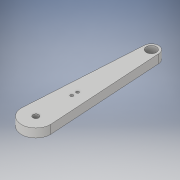
# Autodesk Inventor part: Servo_Arm
Saved by Autodesk Inventor 2019 (Build 230136000, 136)
## iProperties
Created: 2019-09-26
Part Number: Servo_Arm
Material: Generic
Document SubType Name: Modeling
Designer: Jorian Bruslind
Density: 1 g/cm^3
Appearance: Default
Author: Jorian Bruslind
Autodesk Inventor part; units mm, degrees
ref_plane "YZ Plane" through (0, 0, 0) normal (1, 0, 0) x (0, 1, 0)
ref_plane "XZ Plane" through (0, 0, 0) normal (0, 1, 0) x (-1, 0, 0)
ref_plane "XY Plane" through (0, 0, 0) normal (0, 0, 1) x (1, 0, 0)
sketch "Sketch1" plane through (0, 0, 0) normal (0, 1, 0) x (-1, 0, 0)
  circle A0 centre (0, 0) radius 5
  line L0 (0, 0) -> (0, -40)
  circle A1 centre (0, -40) radius 1.75
  circle A2 centre (0, -40) radius 2.5
  line L1 (0, -40) -> (2.5, -40)
  line L2 (0, 0) -> (5, 0)
  line L3 (5, 0) -> (2.5, -40)
  line L4 (0, 0) -> (-5, 0)
  line L5 (0, -40) -> (-2.5, -40)
  line L6 (-5, 0) -> (-2.5, -40)
  dimension "d0" = 10
  dimension "d1" = 40
  dimension "d2" = 3.5
  dimension "d3" = 5
  constraints: 14 end point, 4 point on circle, 3 centre point, 3 coincident, 2 horizontal, 2 parallel, 1 vertical
  measures "d0" diameter of A0
  measures "d1" distance of L0.start L0.end
  measures "d2" diameter of A1
  measures "d3" diameter of A2
extrude "Extrusion1" add sketch "Sketch1" along normal blind 3 contours L2 L4 A0 | L3 A0 L0 L2 | L4 L0 A0 L6 | L3 A2 L0 A0 | A0 L0 A2 L6 | L1 A1 L0 A2 | A2 L5 A1 L1 | A2 L0 A1 L5 | L1 L0 A1 | A1 L5 L1 | A1 L0 L5
sketch "Sketch2" plane through (0, 3, 0) normal (0, 1, 0) x (1, 0, 0)
  arc A0 (2.5, 40) -> (-2.5, 40) centre (0, 40) ccw projected
  circle A1 centre (0, 40) radius 1.75
  point P0 (0, 0)
  dimension "d6" = 3.5
  constraints: 1 centre point, 1 coincident
  measures "d6" diameter of A1
extrude "Extrusion2" cut sketch "Sketch2" against normal blind 5
sketch "Sketch4" plane through (0, 0, 0) normal (0, -1, 0) x (1, 0, 0)
  circle A0 centre (0, 0) radius 4
  line L0 (0, 0) -> (0, -14.45)
  circle A1 centre (0, -14.45) radius 2.5
  line L1 (0, 0) -> (-4, 0)
  line L2 (0, -14.45) -> (-2.5, -14.45)
  line L3 (0, -14.45) -> (2.5, -14.45)
  line L4 (0, 0) -> (4, 0)
  line L5 (2.5, -14.45) -> (13.578, -14.45) construction
  line L6 (2.5, -14.45) -> (3.0315, -2.6097)
  line L7 (2.5, -14.45) -> (14.3523, -14.45) construction
  line L8 (-2.5, -14.45) -> (-3.0325, -2.6084)
  line L9 (-2.5, -14.45) -> (9.3536, -14.45) construction
  dimension "d12" = 8
  dimension "d13" = 14.45
  dimension "d14" = 5
  dimension "d16" = 87.43
  dimension "d17" = 92.575
  constraints: 20 end point, 6 point on circle, 4 horizontal, 2 centre point, 2 coincident, 2 equal length, 2 point on line, 1 parallel, 1 vertical
  measures "d12" diameter of A0
  measures "d13" distance of L0.start L0.end
  measures "d14" diameter of A1
  measures "d16" angle of L7 L6
  measures "d17" angle of L9 L8
extrude "Extrusion4" cut sketch "Sketch4" against normal blind 1.5
sketch "Sketch5" plane through (0, 1.5, 0) normal (0, -1, 0) x (1, 0, 0)
  line L0 (0, 0) -> (0, -14.45)
  circle A0 centre (0, -14.45) radius 0.5
  line L1 (0, -14.45) -> (0, -12.45)
  circle A1 centre (0, -12.45) radius 0.5
  dimension "d20" = 14.45
  dimension "d21" = 1
  dimension "d24" = 2
  dimension "d25" = 1
  constraints: 4 end point, 2 centre point, 2 coincident, 1 point on line, 1 vertical
  measures "d20" distance of L0.start L0.end
  measures "d21" diameter of A0
  measures "d24" distance of L1.start L1.end
  measures "d25" diameter of A1
extrude "Extrusion6" cut sketch "Sketch5" against normal blind 5
sketch "Sketch6" plane through (0, 1.5, 0) normal (0, -1, 0) x (1, 0, 0)
  arc A0 (3.0315, -2.6097) -> (-3.0325, -2.6084) centre (0, 0) ccw projected
  circle A1 centre (0, 0) radius 1
  point P0 (0, 0)
  dimension "d28" = 2
  constraints: 1 centre point, 1 coincident
  measures "d28" diameter of A1
extrude "Extrusion7" cut sketch "Sketch6" against normal blind 2
body "Solid1"
